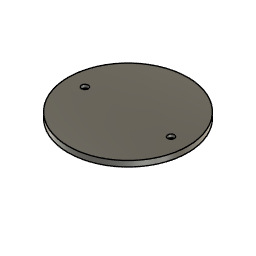
teline rungon kanteen v1 (Autodesk Fusion 360 design; units mm, degrees)
Autodesk Fusion 360 part; units mm, degrees
sketch "Sketch1" plane through (0, 0, 0) normal (0, 0, 1) x (1, 0, 0)
  circle A0 centre (0, 0) radius 31.9
  line L0 (0, 0) -> (-31.9, 0) construction
  line L1 (0, 0) -> (31.9, 0) construction
  circle A1 centre (23.029, 0) radius 1.75
  circle A2 centre (-23.029, 0) radius 1.75
  circle A3 centre (-23.029, 0) radius 3
  circle A4 centre (23.029, 0) radius 3
  circle A5 centre (0, 0) radius 4
  dimension "d1" = 63.8
  dimension "d2" = 3.5
  dimension "d3" = 23.029
  dimension "d4" = 3.5
  dimension "d5" = 23.029
  dimension "d6" = 6
  dimension "d7" = 6
  dimension "d8" = 8
  constraint coincident A0.centre L0.start
  constraint coincident A0 L0.end
  constraint horizontal L0
  constraint coincident A0 L1.end
  constraint parallel L0 L1
  constraint coincident L1 A1.centre
  constraint coincident L0 A2.centre
  constraint concentric A2 A3
  constraint concentric A1 A4
  measures "d1" diameter of A0
  measures "d2" diameter of A1
  measures "d3" distance of A0.centre A1.centre
  measures "d4" diameter of A2
  measures "d5" distance of A0.centre A2.centre
  measures "d6" diameter of A3
  measures "d7" diameter of A4
  measures "d8" diameter of A5
extrude "Extrude1" add sketch "Sketch1" along normal blind 3 contours A0 | A3 | A4 | A5
extrude "Extrude3" add sketch "Sketch1" against normal blind 12 contours A5
fillet "Fillet2" radius 3 1 edges at (-3.7293, -1.4465, 0)
chamfer "Chamfer2" distance 1.25 angle 45 2 edges at (21.3974, 0.6328, 0) (-24.6606, 0.6328, 0)
